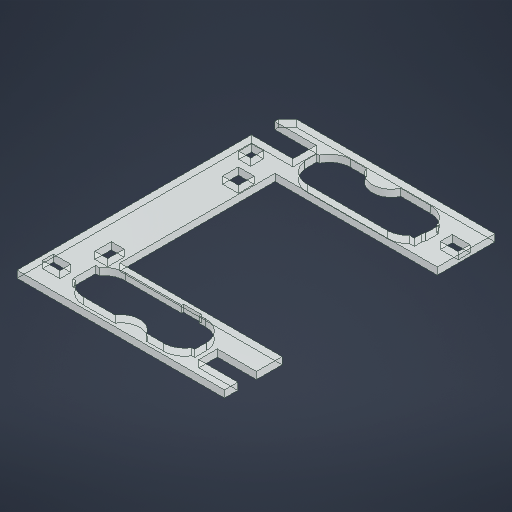
# Autodesk Inventor part: Flex Holder V1
Saved by Autodesk Inventor 2026.2 (Build 302298010, 298A)
## iProperties
Created: 2025-07-01
Part Number: Flex Holder V1
Material: Thermoplastic Resin
Document SubType Name: Modeling
Designer: Caleb Fangmeier
Density: 1.28 g/cm^3
Appearance: Clear
Author: Caleb Fangmeier
Autodesk Inventor part; units mm, degrees
ref_plane "YZ Plane" through (0, 0, 0) normal (1, 0, 0) x (0, 1, 0)
ref_plane "XZ Plane" through (0, 0, 0) normal (0, 1, 0) x (-1, 0, 0)
ref_plane "XY Plane" through (0, 0, 0) normal (0, 0, 1) x (1, 0, 0)
sketch "Sketch1" plane through (0, 0, 0) normal (0, 1, 0) x (-1, 0, 0)
  line L0 (-22.05, -28.75) -> (22.05, -28.75)
  line L1 (22.05, -28.75) -> (22.05, 28.75)
  line L2 (22.05, 28.75) -> (-22.05, 28.75)
  line L3 (-22.05, 28.75) -> (-22.05, -28.75)
  line L4 (-22.05, -28.75) -> (22.05, 28.75) construction
  line L5 (22.05, -28.75) -> (-22.05, 28.75) construction
  point P0 (0, 0)
  dimension "d0" = 57.5
  dimension "d1" = 44.1
  constraints: 12 end point, 2 midpoint, 2 parallel, 1 horizontal, 1 perpendicular
  measures "d0" distance of L0.end L1.end
  measures "d1" distance of L1.end L2.end
extrude "Extrusion1" add sketch "Sketch1" along normal blind 1.5
chamfer "Chamfer1" distance 2 angle 45 1 edges at (-22.05, 0.75, -28.75)
sketch "Sketch4" plane through (0, 1.5, 0) normal (0, 1, 0) x (1, 0, 0)
  line L0 (22.6381, -25.9185) -> (13.7388, -25.9185)
  line L1 (13.7388, -25.9185) -> (13.7388, -21.956)
  line L2 (13.7388, -21.956) -> (22.6381, -21.956)
  line L3 (22.6381, -21.956) -> (22.6381, -25.9185)
  line L4 (11.4165, -21.956) -> (0.7633, -21.956)
  line L5 (0.7633, -21.956) -> (0.7633, -24.4569)
  line L6 (0.7633, -24.4569) -> (11.4165, -24.4569)
  line L7 (11.4165, -24.4569) -> (11.4165, -21.956)
  line L8 (-0.6658, -26.6006) -> (-6.707, -26.6006)
  line L9 (-6.707, -26.6006) -> (-6.707, -22.3783)
  line L10 (-6.707, -22.3783) -> (-0.6658, -22.3783)
  line L11 (-0.6658, -22.3783) -> (-0.6658, -26.6006)
  line L12 (-6.707, -24.392) -> (-14.5426, -24.392)
  line L13 (-14.5426, -24.392) -> (-14.5426, -21.0953)
  line L14 (-14.5426, -21.0953) -> (-6.707, -21.0953)
  line L15 (-6.707, -21.0953) -> (-6.707, -24.392)
  line L16 (-14.5426, -21.0953) -> (-11.8996, -21.0953)
  line L17 (-11.8996, -21.0953) -> (-11.8996, -19.5363)
  line L18 (-11.8996, -19.5363) -> (-14.5426, -19.5363)
  line L19 (-14.5426, -19.5363) -> (-14.5426, -21.0953)
  line L20 (-21.1238, -24.2621) -> (-17.4211, -24.2621)
  line L21 (-17.4211, -24.2621) -> (-17.4211, -21.956)
  line L22 (-17.4211, -21.956) -> (-21.1238, -21.956)
  line L23 (-21.1238, -21.956) -> (-21.1238, -24.2621)
  line L24 (5.6616, -20.7705) -> (1.894, -20.7705)
  line L25 (1.894, -20.7705) -> (1.894, -17.3277)
  line L26 (1.894, -17.3277) -> (5.6616, -17.3277)
  line L27 (5.6616, -17.3277) -> (5.6616, -20.7705)
  line L28 (-2.848, -19.9261) -> (-5.2515, -19.9261)
  line L29 (-5.2515, -19.9261) -> (-5.2515, -18.3346)
  line L30 (-5.2515, -18.3346) -> (-2.848, -18.3346)
  line L31 (-2.848, -18.3346) -> (-2.848, -19.9261)
  line L32 (-17.2689, -17.0029) -> (-14.5426, -17.0029)
  line L33 (-14.5426, -17.0029) -> (-14.5426, -13.4952)
  line L34 (-14.5426, -13.4952) -> (-17.2689, -13.4952)
  line L35 (-17.2689, -13.4952) -> (-17.2689, -17.0029)
  line L36 (15.925, -11.4814) -> (12.4173, -11.4814)
  line L37 (12.4173, -11.4814) -> (12.4173, -14.7294)
  line L38 (12.4173, -14.7294) -> (15.925, -14.7294)
  line L39 (15.925, -14.7294) -> (15.925, -11.4814)
  line L40 (-2.1335, 9.0455) -> (1.894, 9.0455)
  line L41 (1.894, 9.0455) -> (1.894, -8.9481)
  line L42 (1.894, -8.9481) -> (-2.1335, -8.9481)
  line L43 (-2.1335, -8.9481) -> (-2.1335, 9.0455)
  line L44 (4.5573, 3.3291) -> (1.6991, 3.3291)
  line L45 (1.6991, 3.3291) -> (1.6991, 0.6009)
  line L46 (1.6991, 0.6009) -> (4.5573, 0.6009)
  line L47 (4.5573, 0.6009) -> (4.5573, 3.3291)
  line L48 (-17.5287, 13.7631) -> (-14.1519, 13.7631)
  line L49 (-14.1519, 13.7631) -> (-14.1519, 10.4096)
  line L50 (-14.1519, 10.4096) -> (-17.5287, 10.4096)
  line L51 (-17.5287, 10.4096) -> (-17.5287, 13.7631)
  line L52 (16.8052, 16.3739) -> (14.7212, 16.3739)
  line L53 (14.7212, 16.3739) -> (14.7212, 12.4259)
  line L54 (14.7212, 12.4259) -> (16.8052, 12.4259)
  line L55 (16.8052, 12.4259) -> (16.8052, 16.3739)
  line L56 (-23.3919, 26.0219) -> (-13.2211, 26.0219)
  line L57 (-13.2211, 26.0219) -> (-13.2211, 21.0711)
  line L58 (-13.2211, 21.0711) -> (-23.3919, 21.0711)
  line L59 (-23.3919, 21.0711) -> (-23.3919, 26.0219)
  line L60 (-20.3793, 16.7032) -> (-17.8455, 16.7032)
  line L61 (-17.8455, 16.7032) -> (-17.8455, 19.4346)
  line L62 (-17.8455, 19.4346) -> (-20.3793, 19.4346)
  line L63 (-20.3793, 19.4346) -> (-20.3793, 16.7032)
  line L64 (-11.5832, 21.8169) -> (-0.7032, 21.8169)
  line L65 (-0.7032, 21.8169) -> (-0.7032, 24.5446)
  line L66 (-0.7032, 24.5446) -> (-11.5832, 24.5446)
  line L67 (-11.5832, 24.5446) -> (-11.5832, 21.8169)
  line L68 (-2.5673, 18.6812) -> (-4.8458, 18.6812)
  line L69 (-4.8458, 18.6812) -> (-4.8458, 22.2038)
  line L70 (-4.8458, 22.2038) -> (-2.5673, 22.2038)
  line L71 (-2.5673, 22.2038) -> (-2.5673, 18.6812)
  line L72 (0.9146, 27.1153) -> (6.539, 27.1153)
  line L73 (6.539, 27.1153) -> (6.539, 22.2038)
  line L74 (6.539, 22.2038) -> (0.9146, 22.2038)
  line L75 (0.9146, 22.2038) -> (0.9146, 27.1153)
  line L76 (2.2307, 17.9158) -> (4.5573, 17.9158)
  line L77 (4.5573, 17.9158) -> (4.5573, 22.2038)
  line L78 (4.5573, 22.2038) -> (2.2307, 22.2038)
  line L79 (2.2307, 22.2038) -> (2.2307, 17.9158)
  line L80 (6.0899, 24.1958) -> (14.5454, 24.1958)
  line L81 (14.5454, 24.1958) -> (14.5454, 21.5323)
  line L82 (14.5454, 21.5323) -> (6.0899, 21.5323)
  line L83 (6.0899, 21.5323) -> (6.0899, 24.1958)
  line L84 (14.2886, 21.5323) -> (11.9019, 21.5323)
  line L85 (11.9019, 21.5323) -> (11.9019, 19.3557)
  line L86 (11.9019, 19.3557) -> (14.2886, 19.3557)
  line L87 (14.2886, 19.3557) -> (14.2886, 21.5323)
  line L88 (21.4363, 24.0758) -> (17.64, 24.0758)
  line L89 (17.64, 24.0758) -> (17.64, 21.5323)
  line L90 (17.64, 21.5323) -> (21.4363, 21.5323)
  line L91 (21.4363, 21.5323) -> (21.4363, 24.0758)
  point P0 (0, 0)
  point P1 (6.539, 24.1958)
  point P2 (6.0899, 22.2038)
  constraints: 184 end point, 46 parallel, 23 perpendicular, 22 horizontal, 3 point on line
extrude "Clearance Cutouts" cut sketch "Sketch4" against normal blind 1.5
sketch "Sketch5" plane through (0, 1.5, 0) normal (0, 1, 0) x (1, 0, 0)
  line L0 (9.9457, 22.5156) -> (-6.9835, 22.5156) construction
  line L1 (9.9457, 17.9158) -> (-6.9835, 17.9158)
  line L2 (-6.9835, 27.1153) -> (9.9457, 27.1153)
  arc A0 (9.9457, 17.9158) -> (9.9457, 27.1153) centre (9.9457, 22.5156) ccw
  arc A1 (-6.9835, 27.1153) -> (-6.9835, 17.9158) centre (-6.9835, 22.5156) ccw
  line L3 (-11.5832, 24.5446) -> (-0.7032, 24.5446) projected
  line L4 (0.9146, 22.2038) -> (0.9146, 27.1153) projected
  line L5 (-13.2211, 26.0219) -> (-13.2211, 21.0711) projected
  line L6 (-11.5832, 21.8169) -> (-11.5832, 24.5446) projected
  line L7 (14.5454, 24.1958) -> (14.5454, 21.5323) projected
  line L8 (-10.0926, -22.1506) -> (6.9665, -22.1506) construction
  line L9 (-10.0926, -26.6006) -> (6.9665, -26.6006)
  line L10 (6.9665, -17.7006) -> (-10.0926, -17.7006)
  arc A2 (-10.0926, -17.7006) -> (-10.0926, -26.6006) centre (-10.0926, -22.1506) ccw
  arc A3 (6.9665, -26.6006) -> (6.9665, -17.7006) centre (6.9665, -22.1506) ccw
  point P0 (0, 0)
  point P1 (1.4811, 22.5156)
  point P2 (14.5454, 22.5156)
  point P3 (-11.5832, 22.5156)
  point P4 (4.5573, 17.9158)
  point P5 (-1.5631, -22.1506)
  point P6 (-0.6658, -26.6006)
  point P7 (11.4165, -22.1506)
  point P8 (11.4165, -24.4569)
  point P9 (-14.5426, -22.1506)
  point P10 (-14.5426, -19.5363)
  dimension "d53" = 8.9
  constraints: 16 end point, 12 point on circle, 8 tangent, 5 point on line, 4 centre point, 2 horizontal, 2 midpoint, 2 parallel, 2 vertical alignment
  measures "d53" distance between parallel lines of L10 L9
extrude "Extrusion4" cut sketch "Sketch5" against normal blind 1.5 contours L1 A1 L2 A0 | A2 L10 A3 L9
sketch "Sketch6" plane through (0, 0, 0) normal (0, -1, 0) x (1, 0, 0)
  line L0 (22.05, 21.956) -> (22.05, -28.75) projected
  line L1 (22.05, -16.5) -> (-12.45, -16.5)
  line L2 (-12.45, -16.5) -> (-12.45, 16.5)
  line L3 (-12.45, 16.5) -> (22.05, 16.5)
  line L4 (22.05, 16.5) -> (22.05, -16.5)
  point P0 (0, 0)
  point P1 (22.05, 16.5)
  dimension "d44" = 33
  dimension "d45" = 34.5
  dimension "d46" = 16.5
  constraints: 8 end point, 2 parallel, 1 horizontal, 1 perpendicular, 1 point on line
  measures "d44" distance of L1.end L2.end
  measures "d45" distance of L1.start L1.end
  measures "d46" distance from line of L1 point (0, 0)
extrude "Extrusion5" cut sketch "Sketch6" against normal through all
sketch "Sketch7" plane through (0, 1.5, 0) normal (0, 1, 0) x (1, 0, 0)
  line L0 (-22.05, -28.75) -> (22.05, -28.75) projected
  arc A0 (4, -28.75) -> (-4, -28.75) centre (0, -28.75) ccw
  line L1 (22.05, 28.75) -> (-20.05, 28.75) projected
  arc A1 (-4, 28.75) -> (4, 28.75) centre (0, 28.75) ccw
  line L2 (22.05, 28.75) -> (-20.05, 28.75) projected
  point P0 (0, 0)
  point P1 (4, 28.75)
  dimension "d49" = 4
  dimension "d50" = 4
  constraints: 4 point on circle, 4 point on line, 2 centre point, 1 midpoint, 1 vertical alignment
  measures "d49" radius of A0
  measures "d50" radius of A1
extrude "Extrusion6" add sketch "Sketch7" against normal up to surface (1.5 mm away)
equation "\"d46\" = 0.5 * d44"
equation "\"d50\" = d49"
body "Solid1"
